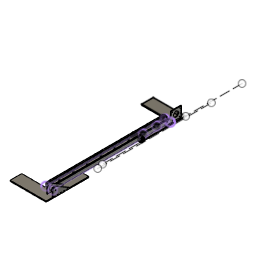
rail (Autodesk Fusion 360 design; units mm, degrees)
Autodesk Fusion 360 part; units mm, degrees
note: some values were not read from the file. Set by a fixed rule: which sketch regions a step uses.
sketch "Sketch1" plane through (0, 0, 0) normal (0, 0, 1) x (1, 0, 0)
  line L0 (-15.05, 0) -> (15.05, 0)
  line L1 (15.05, 0) -> (15.05, 14.6707)
  circle A0 centre (9.55, 11.1) radius 2
  line L2 (9.05, 5) -> (0, 5)
  line L3 (13.929, 15.6634) -> (9.929, 15.1758)
  line L4 (9.05, 14.1831) -> (9.05, 13.0365)
  arc A1 (9.929, 15.1758) -> (9.05, 14.1831) centre (10.05, 14.1831) ccw
  arc A2 (15.05, 14.6707) -> (13.929, 15.6634) centre (14.05, 14.6707) ccw
  line L5 (0, 1.75) -> (0, 22.5)
  line L6 (9.05, 5) -> (9.05, 9.1635)
  line L7 (2.55, 0) -> (9.05, 0)
  line L8 (9.05, 0) -> (9.05, 1)
  line L9 (9.05, 1) -> (2.55, 1)
  line L10 (2.55, 1) -> (2.55, 0)
  line L11 (-9.05, 5) -> (0, 5)
  line L12 (-9.05, 5) -> (-9.05, 9.1635)
  circle A3 centre (-9.55, 11.1) radius 2
  line L13 (-15.05, 0) -> (-15.05, 14.6707)
  arc A4 (-13.929, 15.6634) -> (-15.05, 14.6707) centre (-14.05, 14.6707) ccw
  line L14 (-13.929, 15.6634) -> (-9.929, 15.1758)
  arc A5 (-9.05, 14.1831) -> (-9.929, 15.1758) centre (-10.05, 14.1831) ccw
  line L15 (-2.55, 0) -> (-9.05, 0)
  line L16 (-9.05, 0) -> (-9.05, 1)
  line L17 (-2.55, 1) -> (-2.55, 0)
  line L18 (-9.05, 1) -> (-2.55, 1)
  line L19 (-9.05, 14.1831) -> (-9.05, 13.0365)
  point P0 (15.05, 15.8)
  point P1 (9.05, 15.0686)
  dimension "d1" = 30.1
  dimension "d2" = 15.8
  dimension "d3" = 4
  dimension "d4" = 5
  dimension "d5" = 7.5
  dimension "d6" = 9.1
  dimension "d7" = 6
  dimension "d8" = 2
  dimension "d9" = 1
  dimension "d10" = 6.5
  dimension "d11" = 1
  dimension "d12" = 6
  constraint horizontal L0
  constraint midpoint origin L0
  constraint perpendicular L0 L1
  constraint horizontal L2
  constraint coincident A0 L4.end
  constraint vertical L4
  constraint coincident P1 L3
  constraint coincident P1 L4
  constraint tangent L3 A1
  constraint tangent L4 A1
  constraint coincident P0 L1
  constraint coincident P0 L3
  constraint tangent L1 A2
  constraint tangent L3 A2
  constraint equal A1 A2
  constraint coincident L2.end L5
  constraint vertical L6
  constraint coincident A0 L6.end
  constraint coincident L2.start L6.start
  constraint collinear L4 L6
  constraint horizontal L7
  constraint vertical L8
  constraint horizontal L9
  constraint vertical L10
  constraint coincident L0 L7.start
  constraint symmetric L0.end L5 L0.start
  constraint symmetric A0 L5 A3
  constraint symmetric L2.start L5 L11.start
  constraint symmetric L2.end L5 L11.end
  constraint symmetric L4.end L5 L19.end
  constraint symmetric L3.end L5 L14.end
  constraint symmetric L4.start L5 A5.start
  constraint symmetric A1 L5 A5
  constraint symmetric L1.end L5 L13.end
  constraint symmetric L3.start L5 A4.start
  constraint symmetric A2 L5 A4
  constraint symmetric L5 L2.start L11.start
  constraint symmetric L5 L6.end L12.end
  constraint symmetric L5 L7.start L15.start
  constraint symmetric L5 L7.end L15.end
  constraint symmetric L5 L8.end L16.end
  constraint symmetric L5 L9.end L17.start
  measures "d1" distance of L0.start L0.end
  measures "d2" distance of L0.end P0
  measures "d3" diameter of A0
  measures "d4" distance of L0 L2
  measures "d6" distance of L0 A0
  measures "d7" horizontal distance of P0 P1
  measures "d8" distance of A0 P1
  measures "d9" radius of A1
  measures "d10" distance of L7.start L7.end
  measures "d11" distance of L7.start L9.end
  measures "d12" distance of L1 L8
extrude "Extrude1" add sketch "Sketch1" along normal blind 512 contours L0 L1 A0 L2 L3 L4 A1 A2 L6 L8 L9 L10 L11 L12 A3 L13 A4 L14 A5 L16 L17 L18 L19 | A3 | A0 makes body 1
ref_plane "WorkPlane1" through (0, 7.8589, 256) normal (0, 0, 1) x (1, 0, 0)
sketch "Sketch2" plane through (0, 5, 0) normal (0, 1, 0) x (-1, 0, 0)
  line L0 (-9.05, 0) -> (9.05, 0)
  line L1 (9.05, 0) -> (9.05, 512)
  line L2 (9.05, 512) -> (-9.05, 512)
  line L3 (-9.05, 512) -> (-9.05, 0)
  circle A0 centre (0, 465) radius 3
  line L4 (-9.05, 512) -> (9.05, 512)
  circle A1 centre (0, 465) radius 5
  dimension "d15" = 6
  dimension "d16" = 44
  dimension "d17" = 10
  dimension "d18" = 42
  constraint concentric A0 A1
  measures "d15" diameter of A0
  measures "d16" distance of A0 L4
  measures "d17" diameter of A1
  measures "d18" distance of L4 A1
extrude "Extrude2" cut sketch "Sketch2" against normal through all contours A0 bodies 1
extrude "Extrude3" cut sketch "Sketch2" against normal blind 2.8 contours A1 bodies 1
pattern_linear "R-Pattern1" count 8 spacing 60 along (0, 0, -1) of "Extrude2", "Extrude3"
sketch "Sketch3" plane through (0, 0, 0) normal (0, -1, 0) x (1, 0, 0)
  arc A0 (2.55, 406.5803) -> (-2.55, 406.5803) centre (0, 405) ccw
  line L0 (2.55, 406.5803) -> (2.55, 463.4197)
  arc A1 (-2.55, 463.4197) -> (2.55, 463.4197) centre (0, 465) ccw
  line L1 (-2.55, 463.4197) -> (-2.55, 406.5803)
  circle A2 centre (0, 405) radius 3
  circle A3 centre (0, 465) radius 3
  line L2 (9.05, 512) -> (-9.05, 512)
  line L3 (15.05, 0) -> (15.05, 512)
  line L4 (-15.05, 0) -> (-15.05, 512)
  line L5 (15.05, 382) -> (-15.05, 382)
  line L6 (15.05, 512) -> (15.05, 517)
  line L7 (15.05, 517) -> (115.05, 517)
  line L8 (115.05, 517) -> (115.05, 567)
  line L9 (115.05, 567) -> (-41.5, 567)
  line L10 (-25.05, 570) -> (-25.05, -70) construction
  line L11 (-17.95, 593.095) -> (-17.95, -90.6788) construction
  circle A4 centre (0, 465) radius 4
  circle A5 centre (0, 405) radius 4
  line L12 (-28.6, 574.9642) -> (-28.6, 356.9884) construction
  line L13 (-31.5, 351.7679) -> (-31.5, 592.0573) construction
  line L14 (-41.5, 382) -> (-41.5, 567)
  line L15 (-41.5, 382) -> (-15.05, 382)
  dimension "d26" = 20
  dimension "d27" = 100
  dimension "d28" = 50
  dimension "d29" = 5
  dimension "d32" = 10
  dimension "d33" = 2.9
  dimension "d36" = 1
  dimension "d37" = 1
  dimension "d86" = 16.45
  constraint coincident L3 L5.start
  constraint coincident L4 L5.end
  constraint perpendicular L4 L5
  constraint coincident L3.end L6.start
  constraint parallel L3 L6
  constraint perpendicular L3 L7
  constraint perpendicular L7 L8
  constraint perpendicular L4 L9
  constraint vertical L11
  constraint concentric A3 A4
  constraint concentric A2 A5
  constraint vertical L12
  constraint coincident L9.end L14.end
  constraint perpendicular L14 L15
  measures "d26" distance of A2 L5
  measures "d27" distance of L6.end L7.end
  measures "d28" distance of L7.end L8.end
  measures "d29" distance of L3.end L6.end
  measures "d32" distance of L4 L10
  measures "d33" distance of L4 L11
  measures "d36" distance of A3 A4
  measures "d37" distance of A2 A5
  measures "d86" distance of L10 L14
extrude "Extrude4" add sketch "Sketch3" along normal blind 4.4 separate body contours L0 L1 A4 A5 | L3 L5 L6 L7 L8 L9 L14 L15 makes body 2
move_body "Move1" bodies 2 to x (-1, 0, 0) y (0, -1, 0) z (0, 0, 1) at (0, 0, 0)
move_body "Align1" bodies 2 to x (1, 0, 0) y (0, 1, 0) z (0, 0, 1) at (0, -4.4, 0)
sketch "Sketch4" plane through (0, 0, 0) normal (0, 1, 0) x (-1, 0, 0)
  circle A0 centre (0, 465) radius 4
  circle A1 centre (0, 405) radius 4
  line L0 (15.05, 382) -> (15.05, 517)
  line L1 (15.05, 517) -> (115.05, 517)
  line L2 (115.05, 517) -> (115.05, 567)
  line L3 (115.05, 567) -> (-41.5, 567)
  line L4 (-41.5, 567) -> (-41.5, 382)
  line L5 (-41.5, 382) -> (15.05, 382)
  line L6 (-15.05, 0) -> (-15.05, 512)
  line L7 (-9.05, 512) -> (9.05, 512)
  line L8 (-17.95, 535.8) -> (-15.05, 535.8)
  line L9 (-15.05, 535.8) -> (-15.05, 435.8)
  line L10 (-15.05, 435.8) -> (-17.95, 435.8)
  line L11 (-17.95, 435.8) -> (-17.95, 535.8)
  dimension "d48" = 23.8
  dimension "d49" = 2.9
  dimension "d50" = 100
  constraint horizontal L8
  constraint vertical L9
  constraint horizontal L10
  constraint vertical L11
  constraint collinear L6 L9
  measures "d48" distance of L7 L8
  measures "d49" distance of L9 L11
  measures "d50" distance of L8.start L10.end
sketch "Sketch5" plane through (0, 0, 0) normal (0, -1, 0) x (1, 0, 0)
  arc A0 (2.55, 46.5803) -> (-2.55, 46.5803) centre (0, 45) ccw
  line L0 (2.55, 46.5803) -> (2.55, 103.4197)
  arc A1 (-2.55, 103.4197) -> (2.55, 103.4197) centre (0, 105) ccw
  line L1 (-2.55, 103.4197) -> (-2.55, 46.5803)
  circle A2 centre (0, 105) radius 3
  circle A3 centre (0, 45) radius 3
  line L2 (15.05, 0) -> (15.05, 512)
  line L3 (-15.05, 0) -> (-15.05, 512)
  line L4 (9.05, 0) -> (-9.05, 0)
  line L5 (-15.05, 128) -> (15.05, 128)
  circle A4 centre (0, 105) radius 4
  circle A5 centre (0, 45) radius 4
  line L6 (-15.05, 0) -> (-15.05, -5)
  line L7 (-15.05, -5) -> (-115.05, -5)
  line L8 (-115.05, -5) -> (-115.05, -55)
  line L9 (-115.05, -55) -> (25.9869, -55)
  line L10 (25.05, -300.7283) -> (25.05, 306.2178) construction
  line L11 (31.05, 332.5756) -> (31.05, -161.5123) construction
  dimension "d51" = 20
  dimension "d52" = 1
  dimension "d53" = 1
  dimension "d54" = 100
  dimension "d56" = 50
  dimension "d57" = 5
  dimension "d58" = 10
  dimension "d59" = 6
  constraint coincident L3 L5.start
  constraint perpendicular L3 L5
  constraint concentric A2 A4
  constraint concentric A3 A5
  constraint vertical L6
  constraint perpendicular L6 L7
  constraint perpendicular L7 L8
  constraint perpendicular L8 L9
  constraint coincident L3.start L6.start
  constraint coincident L2 L5.end
  constraint vertical L10
  constraint vertical L11
  measures "d51" distance of A2 L5
  measures "d52" distance of A2 A4
  measures "d53" distance of A3 A5
  measures "d54" distance of L6.end L7.end
  measures "d56" distance of L7.end L8.end
  measures "d57" distance of L3.start L6.end
  measures "d58" distance of L2 L10.end
  measures "d59" horizontal distance of L10.end L11.start
sketch "Sketch6" plane through (15.05, 0, 0) normal (1, 0, 0) x (0, 0, -1)
  line L0 (0, 0) -> (0, 14.6707)
  line L1 (0, 14.6707) -> (-512, 14.6707)
  line L2 (-512, 14.6707) -> (-512, 0)
  line L3 (-512, 0) -> (0, 0)
  line L4 (-332.5756, 0) -> (161.5123, 0)
  line L5 (0, 0) -> (0, 14.6707)
  line L6 (0, 42) -> (42, 42)
  line L7 (42, 42) -> (42, 0)
  line L8 (42, 0) -> (0, 0)
  line L9 (0, 0) -> (0, 42)
  line L10 (42, 0) -> (0, 42) construction
  line L11 (42, 42) -> (0, 0) construction
  circle A0 centre (5.5, 36.5) radius 1.6
  circle A1 centre (36.5, 36.5) radius 1.6
  circle A2 centre (36.5, 5.5) radius 1.6
  circle A3 centre (5.5, 5.5) radius 1.6
  line L12 (5.5, 36.5) -> (36.5, 36.5) construction
  line L13 (5.5, 36.5) -> (5.5, 5.5) construction
  circle A4 centre (21, 21) radius 11
  line L14 (21, 21) -> (-655.1029, 21) construction
  line L15 (42, 42) -> (44.9, 42)
  line L16 (44.9, 42) -> (44.9, 0)
  line L17 (44.9, 0) -> (42, 0)
  line L18 (42, 0) -> (42, 42)
  line L19 (0, 0) -> (44.9, 0)
  line L20 (44.9, 0) -> (44.9, -4.4)
  line L21 (44.9, -4.4) -> (0, -4.4)
  line L22 (0, -4.4) -> (0, 0)
  circle A5 centre (-526, 21) radius 9
  line L23 (-512, 0) -> (-512, 14.6707)
  circle A6 centre (-526, 21) radius 11.9
  line L24 (0, 0) -> (-512, 0)
  line L25 (-382, -4.4) -> (-567, -4.4)
  line L26 (-537.9, 21) -> (-537.9, -4.4)
  line L27 (-520.05, 31.3057) -> (-465.8269, 0)
  circle A7 centre (-526, 21) radius 2.5
  line L28 (-465.8269, 0) -> (-465.8269, -4.4)
  line L29 (0, 26.6707) -> (-26.6707, 0)
  line L30 (-26.6707, 0) -> (-26.6707, -4.4)
  line L31 (-26.6707, -4.4) -> (0, -4.4)
  dimension "d60" = 42
  dimension "d61" = 42
  dimension "d62" = 3.2
  dimension "d63" = 31
  dimension "d64" = 31
  dimension "d65" = 31
  dimension "d66" = 31
  dimension "d67" = 22
  dimension "d68" = 2.9
  dimension "d69" = 4.4
  dimension "d72" = 18
  dimension "d73" = 5
  dimension "d74" = 2.9
  dimension "d75" = 30
  dimension "d76" = 5
  dimension "d99" = 12
  dimension "d100" = 45
  constraint horizontal L6
  constraint vertical L7
  constraint horizontal L8
  constraint vertical L9
  constraint collinear L4 L8
  constraint collinear L0 L9
  constraint coincident L0.start L3.end
  constraint coincident L10 A0.centre
  constraint coincident L11 A1.centre
  constraint coincident L10 A2.centre
  constraint coincident L11 A3.centre
  constraint equal A2 A3
  constraint equal A1 A2
  constraint equal A0 A1
  constraint coincident A0.centre L12.start
  constraint coincident A1.centre L12.end
  constraint coincident A3.centre L13.end
  constraint perpendicular L12 L13
  constraint midpoint L11 A4.centre
  constraint coincident A4.centre L14.start
  constraint horizontal L14
  constraint horizontal L15
  constraint vertical L16
  constraint horizontal L17
  constraint vertical L18
  constraint coincident L4 L16.end
  constraint horizontal L19
  constraint vertical L20
  constraint horizontal L21
  constraint vertical L22
  constraint collinear L16 L20
  constraint coincident L14 A5.centre
  constraint concentric A5 A6
  constraint coincident L14 L26.start
  constraint coincident A6 L26.start
  constraint coincident L25 L26.end
  constraint tangent A6 L26
  constraint coincident A6 L27.start
  constraint tangent A6 L27
  constraint concentric A5 A7
  constraint coincident L3 L27.end
  constraint coincident L25 L28.end
  constraint perpendicular L25 L28
  constraint coincident L9 L29.start
  constraint coincident L4 L29.end
  constraint perpendicular L21 L30
  constraint perpendicular L22 L31
  measures "d60" distance of L6.start L6.end
  measures "d61" distance of L6.start L0.start
  measures "d62" diameter of A0
  measures "d63" horizontal distance of A0.centre A1.centre
  measures "d64" vertical distance of A0.centre A3.centre
  measures "d65" horizontal distance of A2.centre A3.centre
  measures "d66" vertical distance of A1.centre A2.centre
  measures "d67" diameter of A4
  measures "d68" distance of L16 L18
  measures "d69" distance of L4 L21
  measures "d72" diameter of A5
  measures "d73" distance of A5 L23
  measures "d74" distance of A5 A6
  measures "d75" angle of L25 L27
  measures "d76" diameter of A7
  measures "d99" distance of L1 L29.start
  measures "d100" angle of L24 L29
extrude "Extrude5" add sketch "Sketch6" along normal blind 2.9 separate body contours L0 L1 L3 L4 L5 L9 L24 L29 | L3 L4 L22 L24 L30 L31 | L0 L4 L5 L6 L7 L8 L9 L18 L19 | L4 L8 L17 L19 L20 L21 L22 | L1 L9 L29 | L4 L7 L15 L16 L17 L18 L19 makes body 3
ref_plane "WorkPlane2" through (25.05, 7.3354, 245.6187) normal (1, 0, 0) x (0, 0, -1)
extrude "Extrude6" add sketch "Sketch6" along normal blind 2.9 separate body contours L1 L2 L3 L23 L24 L27 | L1 L2 L3 L23 A6 L24 L25 L26 L27 L28 | A6 | A5 makes body 4
sketch "Sketch7" plane through (25.05, 7.3354, 245.6187) normal (1, 0, 0) x (0, 0, -1)
  circle A0 centre (-280.3813, 13.6646) radius 9
  point P0 (-280.3813, 13.6646)
  dimension "d80" = 18
  constraint coincident P0 A0.centre
  measures "d80" diameter of A0
extrude "Extrude7" add sketch "Sketch7" along normal blind 8.65 from surface at -1.1 separate body makes body 5
ref_plane "WorkPlane3" through (28.275, 21, 526) normal (1, 0, 0) x (0, 0, -1)
sketch "Sketch8" plane through (0, -4.4, 0) normal (0, -1, 0) x (1, 0, 0)
  line L0 (15.05, 537.9) -> (15.05, 465.8269)
  line L1 (15.05, 465.8269) -> (17.95, 465.8269)
  line L2 (17.95, 465.8269) -> (17.95, 537.9)
  line L3 (17.95, 537.9) -> (15.05, 537.9)
  line L4 (17.95, 532.9) -> (15.05, 532.9)
  line L5 (15.05, 532.9) -> (15.05, 527.9)
  line L6 (15.05, 527.9) -> (17.95, 527.9)
  line L7 (17.95, 527.9) -> (17.95, 532.9)
  dimension "d87" = 72.0731
  dimension "d88" = 5
  dimension "d89" = 5
  constraint horizontal L4
  constraint vertical L5
  constraint horizontal L6
  constraint vertical L7
  constraint coincident L0 L5.end
  constraint coincident L2 L4.start
  measures "d87" distance of L1.end L2.end
  measures "d88" distance of L3 L4
  measures "d89" distance of L4 L6
extrude "Extrude8" cut sketch "Sketch8" against normal blind 4.4 contours L0 L2 L4 L5 L6 L7 bodies 4
pattern_linear "R-Pattern2" count 5 spacing 14 along (0, 0, -1) of "Extrude8"
mirror "Mirror1" about plane through (28.275, 21, 526) normal (1, 0, 0) of bodies 4 makes body 6
combine "Combine1" operation cut target body 2 tool bodies 4 6 keep tools
sketch "Sketch9" plane through (17.95, 0, 0) normal (1, 0, 0) x (0, 0, -1)
  line L0 (-471.9, 0) -> (-471.9, -4.4)
  line L1 (-471.9, -4.4) -> (-465.8269, -4.4)
  line L2 (-465.8269, -4.4) -> (-465.8269, 0)
  line L3 (-465.8269, 0) -> (-520.05, 31.3057)
  arc A0 (-520.05, 31.3057) -> (-537.9, 21) centre (-526, 21) ccw
  line L4 (-537.9, 21) -> (-537.9, -4.4)
  line L5 (-537.9, -4.4) -> (-532.9, -4.4)
  line L6 (-532.9, -4.4) -> (-532.9, 0)
  line L7 (-532.9, 0) -> (-527.9, 0)
  line L8 (-527.9, 0) -> (-527.9, -4.4)
  line L9 (-527.9, -4.4) -> (-518.9, -4.4)
  line L10 (-518.9, -4.4) -> (-518.9, 0)
  line L11 (-518.9, 0) -> (-513.9, 0)
  line L12 (-513.9, 0) -> (-513.9, -4.4)
  line L13 (-513.9, -4.4) -> (-504.9, -4.4)
  line L14 (-504.9, -4.4) -> (-504.9, 0)
  line L15 (-504.9, 0) -> (-499.9, 0)
  line L16 (-499.9, 0) -> (-499.9, -4.4)
  line L17 (-499.9, -4.4) -> (-490.9, -4.4)
  line L18 (-490.9, -4.4) -> (-490.9, 0)
  line L19 (-490.9, 0) -> (-485.9, 0)
  line L20 (-485.9, 0) -> (-485.9, -4.4)
  line L21 (-485.9, -4.4) -> (-476.9, -4.4)
  line L22 (-476.9, -4.4) -> (-476.9, 0)
  line L23 (-476.9, 0) -> (-471.9, 0)
  circle A1 centre (-526, 21) radius 2.5
  line L24 (0, 14.6707) -> (-512, 14.6707)
  line L25 (-512, 14.6707) -> (-512, 0)
ref_plane "WorkPlane4" through (-14.05, 15.6707, 256) normal (0, 1, 0) x (-1, 0, 0)
ref_plane "WorkPlane5" through (-14.05, 27.6707, 256) normal (0, 1, 0) x (-1, 0, 0)
sketch "Sketch10" plane through (0, -4.4, 0) normal (0, -1, 0) x (1, 0, 0)
  line L0 (15.05, 26.6707) -> (15.05, -44.9)
  line L1 (15.05, -44.9) -> (17.95, -44.9)
  line L2 (17.95, -44.9) -> (17.95, 26.6707)
  line L3 (17.95, 26.6707) -> (15.05, 26.6707)
  line L4 (17.95, 11.6707) -> (15.05, 11.6707)
  line L5 (15.05, 11.6707) -> (15.05, 1.6707)
  line L6 (15.05, 1.6707) -> (17.95, 1.6707)
  line L7 (17.95, 1.6707) -> (17.95, 11.6707)
  dimension "d101" = 15
  dimension "d102" = 10
  constraint horizontal L4
  constraint vertical L5
  constraint horizontal L6
  constraint vertical L7
  constraint coincident L0 L5.end
  constraint coincident L2 L4.start
  measures "d101" distance of L3 L4
  measures "d102" distance of L4 L6
extrude "Extrude9" cut sketch "Sketch10" against normal blind 4.4 contours L0 L2 L4 L5 L6 L7 bodies 3
pattern_linear "R-Pattern3" count 3 spacing 20 along (0, 0, -1) of "Extrude9"
sketch "Sketch11" plane through (0, 0, -44.9) normal (0, 0, -1) x (-1, 0, 0)
  line L0 (-15.05, -4.4) -> (-15.05, 42)
  line L1 (-15.05, 42) -> (-17.95, 42)
  line L2 (-17.95, 42) -> (-17.95, -4.4)
  line L3 (-17.95, -4.4) -> (-15.05, -4.4)
  line L4 (-15.05, 42) -> (26.95, 0)
  line L5 (26.95, 0) -> (-15.05, 42)
  line L6 (15.05, 0) -> (9.05, 0)
  line L7 (26.95, 0) -> (26.95, -4)
  line L8 (26.95, -4) -> (-17.95, -4.4)
  constraint coincident L0.end L1.start
  constraint coincident L2.end L3.start
extrude "Extrude10" add sketch "Sketch11" against normal blind 2.9 separate body contours L0 L1 L2 L8 | L0 L4 L5 L7 L8 makes body 7
sketch "Sketch12" plane through (-0.0378, -4.2398, 0) normal (-0.008908, -0.99996, 0) x (0, 0, 1)
  line L0 (-44.9, 26.9133) -> (-44.9, -17.9885)
  line L1 (-44.9, -17.9885) -> (-42, -17.9885)
  line L2 (-42, -17.9885) -> (-42, 26.9133)
  line L3 (-42, 26.9133) -> (-44.9, 26.9133)
  line L4 (-44.9, 16.9133) -> (-42, 16.9133)
  line L5 (-42, 16.9133) -> (-42, 11.9133)
  line L6 (-42, 11.9133) -> (-44.9, 11.9133)
  line L7 (-44.9, 11.9133) -> (-44.9, 16.9133)
  dimension "d112" = 10
  dimension "d113" = 5
  constraint horizontal L4
  constraint vertical L5
  constraint horizontal L6
  constraint vertical L7
  constraint coincident L2 L5.end
  constraint coincident L0 L4.start
  measures "d112" distance of L3 L4
  measures "d113" distance of L4 L6
extrude "Extrude11" cut sketch "Sketch12" against normal blind 4.4 contours L0 L2 L4 L5 L6 L7 bodies 7
pattern_linear "R-Pattern4" count 4 spacing 10 along (0.99996, -0.008908, 0) of "Extrude11"
sketch "Sketch13" plane through (17.95, 0, 0) normal (1, 0, 0) x (0, 0, -1)
  line L0 (42, 0.0002) -> (44.9, 0.0002)
  line L1 (44.9, 0.0002) -> (44.9, 42)
  line L2 (44.9, 42) -> (42, 42)
  line L3 (42, 42) -> (42, 0.0002)
  line L4 (42, 32) -> (44.9, 32)
  line L5 (44.9, 32) -> (44.9, 27)
  line L6 (44.9, 27) -> (42, 27)
  line L7 (42, 27) -> (42, 32)
  line L8 (42, 42) -> (44.9, 42)
  dimension "d120" = 10
  dimension "d121" = 5
  constraint horizontal L4
  constraint vertical L5
  constraint horizontal L6
  constraint vertical L7
  constraint coincident L1 L5.end
  constraint coincident L3 L4.start
  measures "d120" distance of L4 L8
  measures "d121" distance of L4.end L5.end
extrude "Extrude12" cut sketch "Sketch13" against normal blind 2.9 contours L1 L3 L4 L5 L6 L7 bodies 7
pattern_linear "R-Pattern5" count 3 spacing 11 along (0, -1, 0) of "Extrude12"
combine "Combine2" operation cut target body 3 tool bodies 7 keep tools
sketch "Sketch14" plane through (0, 0, 0) normal (0, -1, 0) x (1, 0, 0)
  line L0 (17.95, -38.3293) -> (17.95, -28.3293)
  line L1 (17.95, -28.3293) -> (15.05, -28.3293)
  line L2 (15.05, -28.3293) -> (15.05, -38.3293)
  line L3 (15.05, -38.3293) -> (17.95, -38.3293)
  line L4 (-15.05, 0) -> (-15.05, -5)
  line L5 (-15.05, -5) -> (-115.05, -5)
  line L6 (-115.05, -5) -> (-115.05, -55)
  line L7 (-115.05, -55) -> (25.9869, -55)
  line L8 (22.95, -55) -> (22.95, 119)
  line L9 (22.95, 119) -> (-15.05, 119)
  line L10 (-15.05, 119) -> (-15.05, 0)
  line L11 (-15.05, 0) -> (-15.05, 512)
  line L12 (17.95, -28.3293) -> (17.95, -38.3293)
  circle A0 centre (0, 105) radius 4
  circle A1 centre (0, 45) radius 4
  dimension "d128" = 5
  dimension "d129" = 10
  constraint coincident L7 L8.start
  constraint perpendicular L7 L8
  constraint perpendicular L8 L9
  constraint coincident L4.start L10.end
  constraint collinear L10 L11
  measures "d128" distance of L8 L12
  measures "d129" distance of L9 A0
extrude "Extrude13" add sketch "Sketch14" along normal blind 4.4 separate body contours L0 L1 L2 L3 L12 | L4 L5 L6 L7 L8 L9 L10 L11 makes body 8
combine "Combine3" operation cut target body 8 tool bodies 7 3 keep tools
equation "d33 = mdfT"
equation "mdfT = 2.9 mm"
equation "idlerT = 8.65 mm"
equation "d37 = d36"
equation "pohjaT = 4.4 mm"
equation "d42 = pohjaT"
equation "idlerOD = 18 mm"
equation "d48 = idlerOD + 2 * mdfT"
equation "d49 = mdfT"
equation "d51 = d26"
equation "d52 = d36"
equation "d53 = d36"
equation "d54 = d27"
equation "d56 = d28"
equation "d57 = d29"
equation "d64 = d63"
equation "d65 = d63"
equation "d68 = mdfT"
equation "d69 = pohjaT"
equation "d70 = mdfT"
equation "d72 = idlerOD"
equation "d74 = mdfT"
equation "d78 = mdfT"
equation "d80 = idlerOD"
equation "d81 = idlerT"
equation "d90 = -pohjaT"
equation "d103 = -pohjaT"
equation "d109 = -mdfT"
equation "d114 = -pohjaT"
equation "d122 = -mdfT"
equation "d130 = pohjaT"
named bodies: "kisko"
